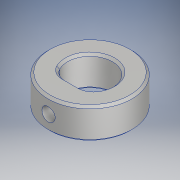
# Autodesk Inventor part: Spacer
Saved by Autodesk Inventor 2019 (Build 230136000, 136)
## iProperties
Created: 2016-04-18
Part Number: Spacer
Material: Aluminum 6061
Document SubType Name: Modeling
Designer: IEUser
Density: 2.7 g/cm^3
Appearance: Aluminum - Flat
Author: IEUser
Autodesk Inventor part; units mm, degrees
note: some values were not read from the file. Chosen so that the rebuilt part matches the saved one: direction of "Cable Hole".
ref_plane "XZ Plane" through (0, 0, 0) normal (0, 1, 0) x (-1, 0, 0)
ref_plane "XY Plane" through (0, 0, 0) normal (0, 0, 1) x (1, 0, 0)
sketch "Body Cross Section" plane through (0, 0, 0) normal (0, 1, 0) x (-1, 0, 0)
  circle A0 centre (0, 0) radius 9.5
  arc A1 (4.05, 3.0996) -> (4.05, -3.0996) centre (0, 0) ccw
  line L0 (4.05, -3.0996) -> (4.05, 3.0996)
  dimension "d0" = 19
  dimension "d1" = 10.2
  dimension "d2" = 4.05
  constraints: 2 centre point, 2 coincident, 2 end point, 2 point on circle, 1 vertical
  measures "d0" diameter of A0
  measures "d1" diameter of A1
  measures "d2" distance from line of point (0, 0) L0
extrude "Body" add sketch "Body Cross Section" along normal mid plane 7
ref_plane "Hole Work Plane" through (-20, 0, 0) normal (1, 0, 0) x (0, 1, 0)
sketch "Cable Hole Position" plane through (-20, 0, 0) normal (1, 0, 0) x (0, 1, 0)
  point P0 (0, 0)
  point P1 (0, 0)
  constraints: 1 coincident
hole "Cable Hole" at (-20, 0, 0) direction (1, 0, 0) diameter 3 end up to surface
fillet "Internal Fillet" radius 3.15 2 edges at (-4.05, 0, -3.0996) (-4.05, 0, 3.0996)
chamfer "Safety Chamfer" distance 0.5 angle 45 10 edges at (-3.5928, 3.5, 3.3643) (5.1, 3.5, 0) (-3.5928, 3.5, -3.3643) (-4.05, 3.5, 0) (5.1, -3.5, 0) (-3.5928, -3.5, -3.3643) (-4.05, -3.5, 0) (-3.5928, -3.5, 3.3643) (9.5, 3.5, 0) (9.5, -3.5, 0)
body "Solid1"
